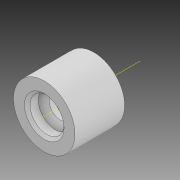
# Autodesk Inventor part: leur adapter2
Saved by Autodesk Inventor 2020 (Build 240168000, 168)
## iProperties
Created: 2020-08-02
Part Number: leur adapter2
Material: Generic
Document SubType Name: Modeling
Designer: DDeGo
Density: 1 g/cm^3
Appearance: Default
Author: DDeGo
Autodesk Inventor part; units mm, degrees
ref_plane "YZ Plane" through (0, 0, 0) normal (1, 0, 0) x (0, 1, 0)
ref_plane "XZ Plane" through (0, 0, 0) normal (0, 1, 0) x (-1, 0, 0)
ref_plane "XY Plane" through (0, 0, 0) normal (0, 0, 1) x (1, 0, 0)
sketch "Sketch1" plane through (0, 0, 0) normal (1, 0, 0) x (0, 1, 0)
  line L0 (0, 0) -> (3.05, 0) construction
  line L1 (5.5, 0) -> (5.5, -8.8811)
  line L2 (5.5, -8.8811) -> (3.5, -8.8811)
  line L3 (3.5, -8.8811) -> (3.5, -3.8811)
  line L4 (3.5, -3.8811) -> (2, -3.8811)
  line L5 (2, -3.8811) -> (2, -2.8811)
  line L6 (2, -2.8811) -> (3.05, -2.8811) construction
  line L7 (3.05, -2.8811) -> (3.05, -2) construction
  line L8 (3.05, 0) -> (5.5, 0)
  line L9 (0, 0) -> (0, -8.8811) construction
  line L10 (0, -8.8811) -> (3.5, -8.8811) construction
  line L11 (2, -2.8811) -> (3.05, -2)
  line L12 (3.05, -2) -> (3.05, 0)
  dimension "d0" = 3.05
  dimension "d3" = 40
  dimension "d4" = 2
  dimension "d5" = 2
  dimension "d6" = 3.5
  dimension "d7" = 2
  dimension "d8" = 5
  dimension "d9" = 1
  constraints: 26 end point, 12 perpendicular, 2 horizontal, 1 vertical
  measures "d0" distance between parallel lines of L9 L7
  measures "d3" angle of L6 L11
  measures "d4" distance between parallel lines of L9 L5
  measures "d5" distance of L7.end L0.end
  measures "d6" distance between parallel lines of L9 L3
  measures "d7" distance between parallel lines of L1 L3
  measures "d8" distance between parallel lines of L4 L2
  measures "d9" distance between parallel lines of L4 L6
revolve "Revolution1" add sketch "Sketch1" angle 360 about axis through (0, 0, 0) along (0, 0, -1)
sketch "Sketch2" plane through (0, 0, 0) normal (0, 1, 0) x (-1, 0, 0)
  line L0 (-3.5, -8.8811) -> (3.5, -8.8811) projected
  line L1 (3.5, -8.8811) -> (3.5, -10.5811)
  line L2 (3.5, -10.5811) -> (4.2, -10.1769)
  line L3 (4.2, -10.1769) -> (4.2, -9.2852)
  line L4 (4.2, -9.2852) -> (3.5, -8.8811)
  point P0 (0, 0)
  dimension "d11" = 0.7
  dimension "d12" = 120
  dimension "d13" = 1.7
  constraints: 8 end point, 1 equal length, 1 parallel, 1 vertical
  measures "d11" distance between parallel lines of L3 L1
  measures "d12" angle of L3 L4
  measures "d13" distance of L0.end L1.end
coil "Coil1" sketch "Sketch2" operation cut axis through (0, 0, -6.3811) along (0, 0, 1) pitch 7 turns 0.857143 hand right
pattern_circular "Circular Pattern1" count 2 over 360 about axis through (0, 0, -6.3811) along (0, 0, -1) of "Coil1"
sketch "Sketch3" plane through (0, 0, -3.8811) normal (0, 0, -1) x (-0.9749279, -0.2225209, 0)
  circle A0 centre (0, 0) radius 5.5 projected
  circle A1 centre (0, 0) radius 2 projected
  point P0 (0, 0)
extrude "Extrusion1" add sketch "Sketch3" against normal blind 1
chamfer "Chamfer1" distance 0.5 angle 45 1 edges at (0, -3.05, 0)
body "Solid1"
